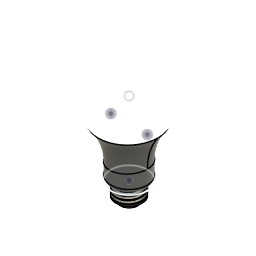
09_DAY- Light Bulb (Autodesk Fusion 360 design; units mm, degrees)
part number: 2025-12-29-13-25-56-661
part number: 2025-12-29-13-26-47-207
Autodesk Fusion 360 part; units mm, degrees
sketch "Sketch1" plane through (0, 0, 0) normal (0, 1, 0) x (1, 0, 0) in component "Bulb"
  circle A0 centre (0, 0) radius 15
  dimension "d1" = 30
  constraint coincident A0.centre origin
  measures "d1" diameter of A0
extrude "Extrude1" add sketch "Sketch1" along normal blind 40 in component "Bulb"
sketch "Sketch2" plane through (0, 0, 0) normal (0, 0, 1) x (1, 0, 0) in component "Bulb"
  line L0 (-15, 40) -> (15, 40) construction
  line L1 (0, 40) -> (0, 60) construction
  point P0 (-15, 40)
  point P1 (15, 40)
  dimension "d4" = 20
  constraint coincident P0 L0.start
  constraint coincident P1 L0.end
  constraint midpoint L0 L1.start
  constraint perpendicular L0 L1
  measures "d4" distance of L1.start L1.end
sphere "SpherePrimitive1" add diameter 61 placed x (1, 0, 0) y (0, 1, 0) z (0, 0, 1) at (-0.9076, 60, 0) in component "Bulb"
fillet "Fillet1" radius 45 1 edges at (-15, 32.9509, 0) in component "Bulb"
fillet "Fillet2" radius 4 1 edges at (-13.9849, 0, 5.4242) in component "Bulb"
sketch "Sketch5" plane through (0, 0, 0) normal (0, -1, 0) x (1, 0, 0) in component "Bulb"
  circle A0 centre (0, 0) radius 11
  circle A1 centre (0, 0) radius 11
  dimension "d10" = 22
  constraint coincident A0.centre A1.centre
  measures "d10" diameter of A1
cylinder "CylinderPrimitive1" add diameter 22 height -15 placed x (1, 0, 0) y (0, 0, -1) z (0, 1, 0) at (0, 0, 0) in component "Bulb"
thread "Thread3" "ANSI Metric M Profile 22.0 M22x3 M22x3 6g" major diameter 21.7645 minor diameter 18.3374 pitch 3 angle 60 modelled right hand crest width 0.4298 on face at (10.8576, -5, 1.7645) from (0, 0, 0) to (0, -11, 0) crest through (0, 0.75, -10.8823) in component "Bulb"
chamfer "Chamfer1" distance 4 angle 45 1 edges at (-3.9352, -15, 10.1458) in component "Bulb"
cylinder "CylinderPrimitive2" add diameter 12 height 2 placed x (1, 0, 0) y (0, 0, 1) z (0, -1, 0) at (0, -15, 0) in component "Bulb"
chamfer "Chamfer2" distance 2 angle 45 1 edges at (-5.594, -17, -2.1697) in component "Bulb"
component "Bulb" placed x (1, 0, 0) y (0, 1, 0) z (0, 0, 1) at (0, 0, 0)
